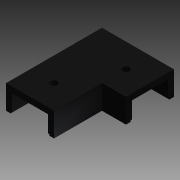
# Autodesk Inventor part: L clamp - top
Saved by Autodesk Inventor 2015 (Build 190159000, 159)
## iProperties
Created: 2013-08-27
Part Number: L clamp - top
Material: PC/ABS Plastic
Document SubType Name: Modeling
Designer: Jesse Stevenson
Density: 0.357273 g/cm^3
Appearance: Glossy - Black
Mass: 3.63067 g
Surface Area: 74.9868 cm^2
Volume: 10.1622 cm^3
Author: Jesse Stevenson
Autodesk Inventor part; units mm, degrees
ref_plane "YZ Plane" through (0, 0, 0) normal (1, 0, 0) x (0, 1, 0)
ref_plane "XZ Plane" through (0, 0, 0) normal (0, 1, 0) x (-1, 0, 0)
ref_plane "XY Plane" through (0, 0, 0) normal (0, 0, 1) x (1, 0, 0)
sketch "Sketch1" plane through (0, 0, 0) normal (0, 0, 1) x (1, 0, 0)
  line L0 (-12.7, -12.7) -> (12.7, -12.7)
  line L1 (12.7, -12.7) -> (12.7, 12.7)
  line L2 (12.7, 12.7) -> (-12.7, 12.7)
  line L3 (-12.7, 12.7) -> (-12.7, -12.7)
  line L4 (-12.7, -12.7) -> (12.7, 12.7) construction
  line L5 (12.7, -12.7) -> (-12.7, 12.7) construction
  point P0 (0, 0)
  dimension "d0" = 25.4
  dimension "d1" = 25.4
  constraints: 12 end point, 2 midpoint, 2 parallel, 1 horizontal, 1 perpendicular
  measures "d0" distance of L2.end L1.end
  measures "d1" distance of L1.end L0.end
extrude "Extrusion1" add sketch "Sketch1" along normal blind 50.8
sketch "Sketch2" plane through (12.7, -12.7, 0) normal (1, 0, 0) x (0, 0, -1)
  line L0 (0, 0) -> (-50.8, 0) projected
  line L1 (0, 25.4) -> (-25.4, 25.4)
  line L2 (-25.4, 25.4) -> (-25.4, 0)
  line L3 (-25.4, 0) -> (0, 0)
  line L4 (0, 0) -> (0, 25.4)
  point P0 (0, 12.7)
  constraints: 8 end point, 2 parallel, 1 horizontal, 1 midpoint, 1 perpendicular
extrude "Extrusion2" add sketch "Sketch2" along normal blind 12.7
sketch "Sketch5" plane through (0, 0, 50.8) normal (0, 0, 1) x (1, 0, 0)
  line L0 (-9.525, 9.525) -> (9.525, 9.525)
  line L1 (9.525, 9.525) -> (9.525, -9.525)
  line L2 (9.525, -9.525) -> (-9.525, -9.525)
  line L3 (-9.525, -9.525) -> (-9.525, 9.525)
  line L4 (-9.525, 9.525) -> (9.525, -9.525) construction
  line L5 (9.525, 9.525) -> (-9.525, -9.525) construction
  point P0 (0, 0)
  dimension "d8" = 19.05
  dimension "d9" = 19.05
  constraints: 12 end point, 2 midpoint, 2 parallel, 1 horizontal, 1 perpendicular
  measures "d8" distance of L1.end L2.end
  measures "d9" distance of L0.end L1.end
extrude "Extrusion4" cut sketch "Sketch5" against normal blind 44.45
sketch "Sketch6" plane through (25.4, -12.7, 0) normal (1, 0, 0) x (0, 0, -1)
  line L0 (-22.225, 22.225) -> (-3.175, 22.225)
  line L1 (-3.175, 22.225) -> (-3.175, 3.175)
  line L2 (-3.175, 3.175) -> (-22.225, 3.175)
  line L3 (-22.225, 3.175) -> (-22.225, 22.225)
  line L4 (-22.225, 22.225) -> (-3.175, 3.175) construction
  line L5 (-3.175, 22.225) -> (-22.225, 3.175) construction
  point P0 (0, 12.7)
  point P1 (-12.7, 12.7)
  dimension "d12" = 19.05
  dimension "d13" = 19.05
  constraints: 12 end point, 2 midpoint, 2 parallel, 1 horizontal, 1 perpendicular
  measures "d12" distance of L1.end L2.end
  measures "d13" distance of L0.end L1.end
extrude "Extrusion5" cut sketch "Sketch6" against normal up to surface (34.925 mm away)
sketch "Sketch7" plane through (-12.7, -12.7, 50.8) normal (0, -1, 0) x (1, 0, 0)
  line L0 (0, -50.8) -> (38.1, -50.8) projected
  line L1 (38.1, -25.4) -> (38.1, -50.8) projected
  line L2 (25.4, -25.4) -> (25.4, 0) projected
  line L3 (0, 0) -> (25.4, 0) projected
  line L4 (0, -50.8) -> (0, 0) projected
  line L5 (-12.7, -50.8) -> (-12.7, -25.4) projected
  line L6 (12.7, -50.8) -> (12.7, 0) construction
  line L7 (-12.7, -38.1) -> (38.1, -38.1) construction
  line L8 (25.4, -25.4) -> (25.4, -50.8) construction
  line L9 (0, -12.7) -> (25.4, -12.7) construction
  circle A0 centre (12.7, -12.7) radius 1.7907
  circle A1 centre (0, -38.1) radius 1.7907
  circle A2 centre (25.4, -38.1) radius 1.7907
  point P0 (0, -25.4)
  dimension "d34" = 3.5814
  constraints: 8 end point, 6 midpoint, 3 centre point, 3 point on line, 2 equal radius, 1 perpendicular
  measures "d34" diameter of A0
extrude "Extrusion6" cut sketch "Sketch7" against normal through all contours A0 | A2
split "Split2" plane through (0, 0, 0) removes the side toward (0, -1, 0)
lip "Lip4" kind groove height 0.762 width 0.762 edges at (9.525, 0, 36.5125) (17.4625, 0, 22.225) guide face at (10.5833, 0, 32.8083)
lip "Lip5" kind groove height 0.762 width 0.762 edges at (-9.525, 0, 26.9875) (7.9375, 0, 3.175) guide face at (-11.6417, 0, 17.9917)
body "Solid1"
